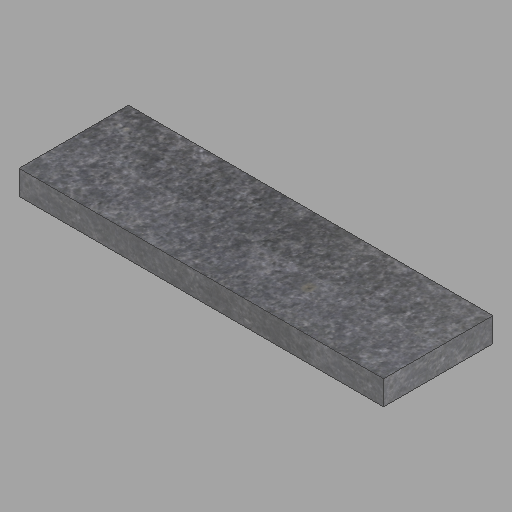
# Autodesk Inventor part: model
Saved by Autodesk Inventor 2022.2 (Build 262287010, 287A)
## iProperties
RuleStatus: InUse
Created: 2022-03-29
Part Number: model
Material: Granite, Cut, Polished
Document SubType Name: Modeling
Designer: awelt
Mass: 191139 g
Surface Area: 17961.3 cm^2
Volume: 70792.1 cm^3
Density: 2.7 g/cm^3
Appearance: Kasota SN sapphire
AfterDocSave0: in3 to ft3 2
in3 to ft3 2: 2.5
TEST: 2.5
Author: awelt
Autodesk Inventor part; units mm, degrees
ref_plane "YZ Plane" through (0, 0, 0) normal (1, 0, 0) x (0, 1, 0)
ref_plane "XZ Plane" through (0, 0, 0) normal (0, 1, 0) x (-1, 0, 0)
ref_plane "XY Plane" through (0, 0, 0) normal (0, 0, 1) x (1, 0, 0)
sketch "Sketch1" plane through (0, 0, 0) normal (0, 1, 0) x (-1, 0, 0)
  line L0 (0, 0) -> (-1524, 0)
  line L1 (-1524, 0) -> (-1524, -457.2)
  line L2 (-1524, -457.2) -> (0, -457.2)
  line L3 (0, -457.2) -> (0, 0)
  dimension "d0" = 1524
  dimension "d1" = 457.2
  constraints: 8 end point, 2 parallel, 1 horizontal, 1 perpendicular
  measures "d0" distance of L2.end L1.end
  measures "d1" distance of L1.end L0.end
extrude "Extrusion1" add sketch "Sketch1" along normal blind 101.6
body "Solid1"
